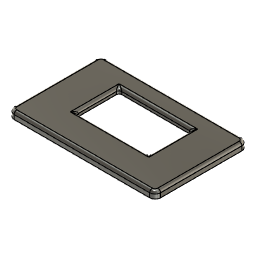
ad_oled_cover (Autodesk Fusion 360 design; units mm, degrees)
Autodesk Fusion 360 part; units mm, degrees
sketch "Sketch1" plane through (0, 0, 0) normal (0, 0, 1) x (1, 0, 0)
  line L0 (0, 0) -> (54, 0)
  line L1 (54, 0) -> (54, 34)
  line L2 (54, 34) -> (0, 34)
  line L3 (0, 34) -> (0, 0)
  line L4 (13.5, 27.2) -> (40.5, 27.2)
  line L5 (40.5, 27.2) -> (40.5, 11.2)
  line L6 (40.5, 11.2) -> (13.5, 11.2)
  line L7 (13.5, 11.2) -> (13.5, 27.2)
  line L8 (12, 31.5) -> (42, 31.5)
  line L9 (42, 31.5) -> (42, 2.5)
  line L10 (42, 2.5) -> (12, 2.5)
  line L11 (12, 2.5) -> (12, 31.5)
  line L12 (54, 29) -> (54, 2)
  line L13 (0, 2) -> (0, 29)
  line L14 (2, 32) -> (52, 32)
  line L15 (52, 32) -> (52, 2)
  line L16 (52, 2) -> (2, 2)
  line L17 (2, 2) -> (2, 32)
  dimension "d9" = 34
  dimension "d10" = 54
  dimension "d11" = 27
  dimension "d12" = 16
  dimension "d14" = 13.5
  dimension "d15" = 30
  dimension "d16" = 29
  dimension "d17" = 12
  dimension "d19" = 4.3
  dimension "d20" = 2.5
  dimension "d33" = 50
  dimension "d34" = 30
  dimension "d35" = 2
  dimension "d36" = 2
  constraint horizontal L0
  constraint vertical L1
  constraint horizontal L2
  constraint vertical L3
  constraint coincident L0.start L3.end
  constraint horizontal L4
  constraint vertical L5
  constraint horizontal L6
  constraint vertical L7
  constraint horizontal L8
  constraint vertical L9
  constraint horizontal L10
  constraint vertical L11
  constraint vertical L12
  constraint vertical L13
  constraint coincident L1 L12.end
  constraint coincident L3 L13.end
  constraint horizontal L14
  constraint vertical L15
  constraint horizontal L16
  constraint vertical L17
  measures "d9" distance of L0.start L2.end
  measures "d10" distance of L1 L3
  measures "d11" distance of L4.start L4.end
  measures "d12" distance of L4.start L6.end
  measures "d14" distance of L1 L5
  measures "d15" distance of L8.start L8.end
  measures "d16" distance of L8.start L10.end
  measures "d17" distance of L1 L9
  measures "d19" distance of L4 L8
  measures "d20" distance of L2 L8
  measures "d33" distance of L14.start L14.end
  measures "d34" distance of L14.start L16.end
  measures "d35" distance of L12 L15
  measures "d36" distance of L2 L14
extrude "Extrude1" add sketch "Sketch1" along normal blind 2.6 contours L0 L1 L2 L3 L12 L13 | L8 L9 L10 L11 | L14 L15 L16 L17
extrude "Extrude2" cut sketch "Sketch1" along normal blind 0.6 contours L8 L9 L10 L11
fillet "Fillet1" radius 1 4 edges at (27, 27.2, 2.6) (13.5, 19.2, 2.6) (27, 11.2, 2.6) (40.5, 19.2, 2.6)
fillet "Fillet2" radius 2 4 edges at (54, 0, 1.3) (54, 34, 1.3) (0, 34, 1.3) (0, 0, 1.3)
fillet "Fillet3" radius 1 8 edges at (0.5858, 0.5858, 2.6) (27, 0, 2.6) (53.4142, 0.5858, 2.6) (54, 17, 2.6) (53.4142, 33.4142, 2.6) (27, 34, 2.6) (0.5858, 33.4142, 2.6) (0, 17, 2.6)
extrude "Extrude3" cut sketch "Sketch1" along normal blind 0.1 contours L4 L5 L6 L7 | L8 L9 L10 L11 | L14 L15 L16 L17
fillet "Fillet4" radius 1 8 edges at (13.5, 11.2, 1.1) (13.2071, 10.9071, 2.3071) (40.5, 11.2, 1.1) (40.7929, 10.9071, 2.3071) (40.5, 27.2, 1.1) (40.7929, 27.4929, 2.3071) (13.5, 27.2, 1.1) (13.2071, 27.4929, 2.3071)
equation "oled_w = 27 mm"
equation "oled_l = 16 mm"
equation "oled_board_w = 30 mm"
equation "oled_board_l = 29 mm"
equation "w = 50 mm"
equation "len = 30 mm"
equation "h = 0.6 mm"
equation "wall = 2 mm"
equation "d9 = len + wall * 2"
equation "d10 = w + wall * 2"
equation "d11 = oled_w"
equation "d12 = oled_l"
equation "d14 = ( w + wall * 2 - oled_w ) / 2"
equation "d15 = oled_board_w"
equation "d16 = oled_board_l"
equation "d17 = ( w + wall * 2 - oled_board_w ) / 2"
equation "oled_b_off = 4.30 mm"
equation "d19 = oled_b_off"
equation "d20 = ( len + wall * 2 - oled_board_l ) / 2"
equation "d21 = h + wall"
equation "d23 = h"
equation "d30 = cut"
equation "cut = 0.1 mm"
equation "d33 = w"
equation "d34 = len"
equation "d35 = wall"
equation "d36 = wall"
named bodies: "ad_oled_cover"
